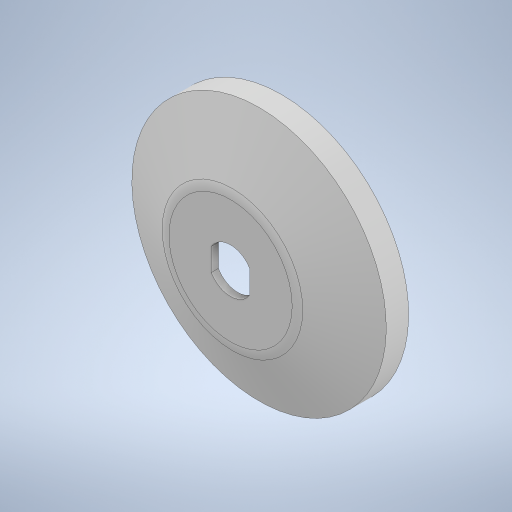
# Autodesk Inventor part: CVT_Ring
Saved by Autodesk Inventor 2023 (Build 270158000, 158)
## iProperties
Created: 2023-07-12
Part Number: CVT_Ring
Material: Generic
Document SubType Name: Modeling
Designer: checo
Density: 1 g/cm^3
Appearance: Default
units: mm
Author: checo
Autodesk Inventor part; units mm, degrees
ref_plane "YZ Plane" through (0, 0, 0) normal (1, 0, 0) x (0, 1, 0)
ref_plane "XY Plane" through (0, 0, 0) normal (0, 0, 1) x (1, 0, 0)
sketch "Sketch1" plane through (0, 0, 0) normal (0, 0, 1) x (1, 0, 0)
  circle A0 centre (0, 0) radius 11
  line L0 (-9.5, 5.5453) -> (-9.5, -5.5453)
  line L1 (9.5, 5.5453) -> (9.5, -5.5453)
  circle A1 centre (0, 0) radius 32.5
  dimension "d0" = 22
  dimension "d1" = 19
  dimension "d2" = 65
  constraints: 4 end point, 4 point on circle, 2 centre point, 2 coincident, 2 parallel, 1 vertical
  measures "d0" diameter of A0
  measures "d1" distance between parallel lines of L1 L0
  measures "d2" diameter of A1
extrude "Extrusion1" add sketch "Sketch1" along normal blind 3.5 contours A0 L1 | L0 A0 | A1
sketch "Sketch2" plane through (0, 0, 0) normal (1, 0, 0) x (0, 1, 0)
  line L0 (32.5, 0) -> (-32.5, 0) projected
  line L1 (32.5, 0) -> (55.5, -21.5)
  line L2 (55.5, -21.5) -> (62.5, -21.5)
  line L3 (62.5, -21.5) -> (62.5, -10.5)
  line L4 (32.5, 3.5) -> (-32.5, 3.5) projected
  line L5 (32.5, 3.5) -> (62.5, -10.5)
  line L6 (0, 0) -> (0, -19.375) construction
  line L7 (32.5, 3.5) -> (32.5, 0)
  dimension "d8" = 7
  dimension "d9" = 25
  dimension "d10" = 11
  dimension "d11" = 30
  constraints: 12 end point, 1 parallel, 1 perpendicular, 1 point on line, 1 vertical
  measures "d8" distance of L1.end L2.end
  measures "d9" distance between parallel lines of L4 L2
  measures "d10" distance of L2.end L3.end
  measures "d11" distance between parallel lines of L7 L3
revolve "Revolution1" add sketch "Sketch2" angle 360 about axis through (0, 0, 0) along (0, 0, -1)
fillet "Fillet1" radius 10 1 edges at (0, -32.5, 3.5)
ref_plane "Work Plane2" through (0, 61, 0) normal (0, 1, 0) x (-1, 0, 0)
sketch "Sketch3" plane through (0, 61, 0) normal (0, 1, 0) x (-1, 0, 0)
  circle A0 centre (0, -16) radius 4.5
  line L0 (4.5, -16) -> (4.5, -20.5)
  line L1 (-4.5, -20.5) -> (-4.5, -16)
  line L2 (-62.5, -21.5) -> (62.5, -21.5) projected
  line L3 (62.5, -21.5) -> (62.5, -11.7) construction
  line L4 (62.5, -10.5) -> (62.5, -21.5) projected
  line L5 (-9.5, 0) -> (9.5, 0) projected
  line L6 (-4.5, -20.5) -> (4.5, -20.5)
  point P0 (0, 0)
  point P1 (0, 0)
  point P2 (0, -20.5)
  dimension "d14" = 9
  dimension "d22" = 1
  constraints: 8 end point, 3 tangent, 2 point on circle, 2 vertical, 1 centre point, 1 horizontal, 1 midpoint, 1 point on line, 1 vertical alignment
  measures "d14" diameter of A0
  measures "d22" distance between parallel lines of L2 L6
extrude "Extrusion2" cut sketch "Sketch3" against normal blind 6
sketch "Sketch4" plane through (0, 0, 3.5) normal (0, 0, 1) x (1, 0, 0)
  circle A0 centre (0, 45) radius 9
  point P0 (0, 0)
  dimension "d25" = 45
  dimension "d26" = 18
  constraints: 1 centre point, 1 vertical alignment
  measures "d25" distance of A0.centre point (0, 0)
  measures "d26" diameter of A0
extrude "Extrusion3" [suppressed]
pattern_circular "Circular Pattern1" [suppressed]
body "Solid1"
